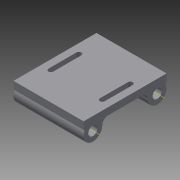
# Autodesk Inventor part: DC Motor stand V2
Saved by Autodesk Inventor 2013 (Build 170138000, 138)
## iProperties
Created: 2013-01-04
Part Number: DC Motor stand V2
Material: Generic
Document SubType Name: Modeling
Designer: Nico
Density: 1 g/cm^3
Author: Nico
Autodesk Inventor part; units mm, degrees
ref_plane "YZ Plane" through (0, 0, 0) normal (1, 0, 0) x (0, 1, 0)
ref_plane "XZ Plane" through (0, 0, 0) normal (0, 1, 0) x (-1, 0, 0)
ref_plane "XY Plane" through (0, 0, 0) normal (0, 0, 1) x (1, 0, 0)
sketch "Sketch1" plane through (0, 0, 0) normal (0, 0, 1) x (1, 0, 0)
  line L0 (0, 0) -> (60, 0)
  line L1 (60, 0) -> (60, 71)
  line L2 (60, 71) -> (0, 71)
  line L3 (0, 71) -> (0, 0)
  dimension "d0" = 60
  dimension "d1" = 71
  constraints: 8 end point, 2 parallel, 1 horizontal, 1 perpendicular
  measures "d0" distance of L0.start L0.end
  measures "d1" distance of L2.end L0.start
extrude "Extrusion1" add sketch "Sketch1" along normal blind 6
sketch "Sketch2" plane through (0, 0, 6) normal (0, 0, 1) x (1, 0, 0)
  line L0 (0, 0) -> (60, 0) projected
  line L1 (0, 71) -> (0, 0) projected
  arc A0 (5.9, 24) -> (10.1, 24) centre (8, 24) ccw
  arc A1 (49.9, 24) -> (54.1, 24) centre (52, 24) ccw
  arc A2 (54.1, 48) -> (49.9, 48) centre (52, 48) ccw
  arc A3 (10.1, 48) -> (5.9, 48) centre (8, 48) ccw
  line L2 (10.1, 48) -> (10.1, 24)
  line L3 (5.9, 24) -> (5.9, 48)
  line L4 (54.1, 48) -> (54.1, 24)
  line L5 (49.9, 24) -> (49.9, 48)
  dimension "d4" = 4.2
  dimension "d6" = 4.2
  dimension "d7" = 4.2
  dimension "d9" = 44
  dimension "d10" = 44
  dimension "d13" = 24
  dimension "d14" = 24
  dimension "d15" = 8
  dimension "d16" = 8
  dimension "d35" = 48
  dimension "d36" = 48
  dimension "d37" = 4.2
  dimension "d38" = 4.2
  dimension "d39" = 2.1
  constraints: 8 end point, 8 point on circle, 4 centre point, 2 parallel
  measures "d4" diameter of A0
  measures "d6" diameter of A1
  measures "d7" diameter of A2
  measures "d9" distance of A2.centre A3.centre
  measures "d10" distance of A1.centre A0.centre
  measures "d13" distance from line of L0 A0.centre
  measures "d14" distance from line of L0 A1.centre
  measures "d15" distance from line of L1 A3.centre
  measures "d16" distance from line of L1 A0.centre
  measures "d35" distance from line of L0 A2.centre
  measures "d36" distance from line of L0 A3.centre
  measures "d37" distance between parallel lines of L3 L2
  measures "d38" distance between parallel lines of L5 L4
  measures "d39" radius of A3
extrude "Extrusion2" cut sketch "Sketch2" against normal blind 6
sketch "Sketch3" plane through (60, 0, 0) normal (1, 0, 0) x (0, 0, -1)
  line L0 (0, 0) -> (0, 71) projected
  circle A0 centre (5, 62.9091) radius 3.9
  circle A1 centre (5, 7.9091) radius 3.9
  circle A2 centre (5, 62.9091) radius 8
  circle A3 centre (5, 7.9091) radius 8
  dimension "d19" = 7.8
  dimension "d21" = 7.8
  dimension "d22" = 55
  dimension "d24" = 16
  dimension "d25" = 16
  dimension "d26" = 5
  dimension "d31" = 5
  constraints: 4 centre point, 2 coincident
  measures "d19" diameter of A0
  measures "d21" diameter of A1
  measures "d22" distance of A1.centre A0.centre
  measures "d24" diameter of A2
  measures "d25" diameter of A3
  measures "d26" distance from line of A0.centre L0
  measures "d31" distance from line of L0 A1.centre
extrude "Extrusion3" add sketch "Sketch3" against normal blind 60
fillet "Fillet1" radius 1 1 edges at (30, 69.1541, 0)
fillet "Fillet2" radius 1 1 edges at (30, 1.6641, 0)
fillet "Fillet3" radius 5 2 edges at (30, 56.6641, 0) (30, 14.1541, 0)
body "Solid1"
